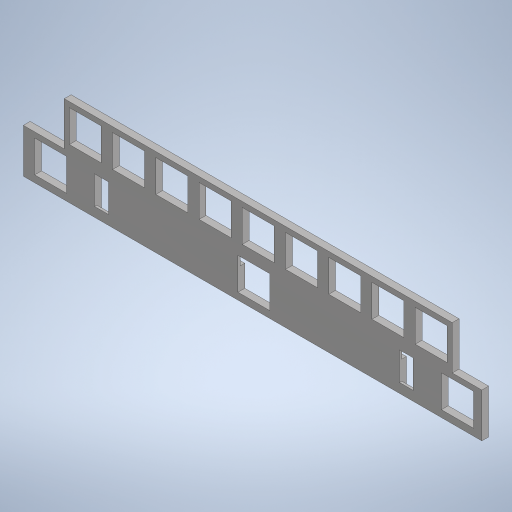
# Autodesk Inventor part: Lower Middle Plate
Saved by Autodesk Inventor 2024 (Build 280153000, 153)
## iProperties
Created: 2024-06-29
Part Number: Lower Middle Plate
Material: PET Plastic
Document SubType Name: Modeling
Designer: adam
Density: 1.541 g/cm^3
Appearance: Light Gray
Author: adam
Autodesk Inventor part; units mm, degrees
ref_plane "YZ Plane" through (0, 0, 0) normal (1, 0, 0) x (0, 1, 0)
ref_plane "XZ Plane" through (0, 0, 0) normal (0, 1, 0) x (-1, 0, 0)
ref_plane "XY Plane" through (0, 0, 0) normal (0, 0, 1) x (1, 0, 0)
sketch "Sketch1" plane through (0, 0, 0) normal (0, 0, 1) x (1, 0, 0)
  line L0 (31.275, 11.925) -> (31.275, -2.125) construction
  line L1 (31.275, -2.125) -> (17.225, -2.125) construction
  line L2 (17.225, -2.125) -> (17.225, 11.925) construction
  line L3 (17.225, 11.925) -> (31.275, 11.925) construction
  line L4 (-101.725, 11.925) -> (-101.725, -2.125) construction
  line L5 (-101.725, -2.125) -> (-115.775, -2.125) construction
  line L6 (-115.775, -2.125) -> (-115.775, 11.925) construction
  line L7 (-115.775, 11.925) -> (-101.725, 11.925) construction
  line L8 (43.325, -43.95) -> (49.375, -43.95) construction
  line L9 (49.375, -43.95) -> (49.375, -61) construction
  line L10 (49.375, -61) -> (43.325, -61) construction
  line L11 (43.325, -61) -> (43.325, -43.95) construction
  line L12 (117.95, -19.8) -> (117.95, -13.75) construction
  line L13 (117.95, -13.75) -> (135, -13.75) construction
  line L14 (135, -13.75) -> (135, -19.8) construction
  line L15 (135, -19.8) -> (117.95, -19.8) construction
  line L16 (26.325, -43.95) -> (32.375, -43.95) construction
  line L17 (32.375, -43.95) -> (32.375, -61) construction
  line L18 (32.375, -61) -> (26.325, -61) construction
  line L19 (26.325, -61) -> (26.325, -43.95) construction
  line L20 (-152.525, 13.425) -> (-146.475, 13.425) construction
  line L21 (-146.475, 13.425) -> (-146.475, -3.625) construction
  line L22 (-146.475, -3.625) -> (-152.525, -3.625) construction
  line L23 (-152.525, -3.625) -> (-152.525, 13.425) construction
  line L24 (-90.675, -43.95) -> (-84.625, -43.95) construction
  line L25 (-84.625, -43.95) -> (-84.625, -61) construction
  line L26 (-84.625, -61) -> (-90.675, -61) construction
  line L27 (-90.675, -61) -> (-90.675, -43.95) construction
  line L28 (39.375, -43.95) -> (39.375, -61) construction
  line L29 (39.375, -61) -> (33.325, -61) construction
  line L30 (33.325, -61) -> (33.325, -43.95) construction
  line L31 (33.325, -43.95) -> (39.375, -43.95) construction
  line L32 (117.95, 4.2) -> (117.95, 10.25) construction
  line L33 (117.95, 10.25) -> (135, 10.25) construction
  line L34 (135, 10.25) -> (135, 4.2) construction
  line L35 (135, 4.2) -> (117.95, 4.2) construction
  line L36 (-67.625, -43.95) -> (-67.625, -61) construction
  line L37 (-67.625, -61) -> (-73.675, -61) construction
  line L38 (-73.675, -61) -> (-73.675, -43.95) construction
  line L39 (-73.675, -43.95) -> (-67.625, -43.95) construction
  line L40 (-128.525, 13.425) -> (-122.475, 13.425) construction
  line L41 (-122.475, 13.425) -> (-122.475, -3.625) construction
  line L42 (-122.475, -3.625) -> (-128.525, -3.625) construction
  line L43 (-128.525, -3.625) -> (-128.525, 13.425) construction
  line L44 (-74.625, -43.95) -> (-74.625, -61) construction
  line L45 (-74.625, -61) -> (-80.675, -61) construction
  line L46 (-80.675, -61) -> (-80.675, -43.95) construction
  line L47 (-80.675, -43.95) -> (-74.625, -43.95) construction
  line L48 (-157.5, -62.5) -> (157.5, -62.5) construction
  line L49 (157.5, -62.5) -> (157.5, -41.5) construction
  line L50 (157.5, -41.5) -> (139.5, -41.5) construction
  line L51 (139.5, -41.5) -> (139.5, 12.5) construction
  line L52 (139.5, 12.5) -> (157.5, 12.5) construction
  line L53 (157.5, 12.5) -> (157.5, 62.5) construction
  line L54 (157.5, 62.5) -> (-157.5, 62.5) construction
  line L55 (-157.5, 62.5) -> (-157.5, -62.5) construction
  line L56 (-38.5, 42.5) -> (6.5, 42.5) construction
  line L57 (6.5, 42.5) -> (6.5, 33.5) construction
  line L58 (6.5, 33.5) -> (-38.5, 33.5) construction
  line L59 (-38.5, 33.5) -> (-38.5, 42.5) construction
  line L60 (154.775, -45.45) -> (154.775, -59.5) construction
  line L61 (154.775, -59.5) -> (140.725, -59.5) construction
  line L62 (140.725, -59.5) -> (140.725, -45.45) construction
  line L63 (140.725, -45.45) -> (154.775, -45.45) construction
  line L64 (135.775, -45.45) -> (135.775, -59.5) construction
  line L65 (135.775, -59.5) -> (121.725, -59.5) construction
  line L66 (121.725, -59.5) -> (121.725, -45.45) construction
  line L67 (121.725, -45.45) -> (135.775, -45.45) construction
  line L68 (116.775, -45.45) -> (116.775, -59.5) construction
  line L69 (116.775, -59.5) -> (102.725, -59.5) construction
  line L70 (102.725, -59.5) -> (102.725, -45.45) construction
  line L71 (102.725, -45.45) -> (116.775, -45.45) construction
  line L72 (97.775, -45.45) -> (97.775, -59.5) construction
  line L73 (97.775, -59.5) -> (83.725, -59.5) construction
  line L74 (83.725, -59.5) -> (83.725, -45.45) construction
  line L75 (83.725, -45.45) -> (97.775, -45.45) construction
  line L76 (75.775, -45.45) -> (75.775, -59.5) construction
  line L77 (75.775, -59.5) -> (61.725, -59.5) construction
  line L78 (61.725, -59.5) -> (61.725, -45.45) construction
  line L79 (61.725, -45.45) -> (75.775, -45.45) construction
  line L80 (-13.625, -45.45) -> (-13.625, -59.5) construction
  line L81 (-13.625, -59.5) -> (-27.675, -59.5) construction
  line L82 (-27.675, -59.5) -> (-27.675, -45.45) construction
  line L83 (-27.675, -45.45) -> (-13.625, -45.45) construction
  line L84 (-102.975, -45.45) -> (-102.975, -59.5) construction
  line L85 (-102.975, -59.5) -> (-117.025, -59.5) construction
  line L86 (-117.025, -59.5) -> (-117.025, -45.45) construction
  line L87 (-117.025, -45.45) -> (-102.975, -45.45) construction
  line L88 (-141.525, -45.45) -> (-127.475, -45.45) construction
  line L89 (-127.475, -45.45) -> (-127.475, -59.5) construction
  line L90 (-127.475, -59.5) -> (-141.525, -59.5) construction
  line L91 (-141.525, -59.5) -> (-141.525, -45.45) construction
  line L92 (121.725, -26.275) -> (135.775, -26.275) construction
  line L93 (135.775, -26.275) -> (135.775, -40.325) construction
  line L94 (135.775, -40.325) -> (121.725, -40.325) construction
  line L95 (121.725, -40.325) -> (121.725, -26.275) construction
  line L96 (95.475, -26.275) -> (109.525, -26.275) construction
  line L97 (109.525, -26.275) -> (109.525, -40.325) construction
  line L98 (109.525, -40.325) -> (95.475, -40.325) construction
  line L99 (95.475, -40.325) -> (95.475, -26.275) construction
  line L100 (69.225, -26.275) -> (83.275, -26.275) construction
  line L101 (83.275, -26.275) -> (83.275, -40.325) construction
  line L102 (83.275, -40.325) -> (69.225, -40.325) construction
  line L103 (69.225, -40.325) -> (69.225, -26.275) construction
  line L104 (50.225, -26.275) -> (64.275, -26.275) construction
  line L105 (64.275, -26.275) -> (64.275, -40.325) construction
  line L106 (64.275, -40.325) -> (50.225, -40.325) construction
  line L107 (50.225, -40.325) -> (50.225, -26.275) construction
  line L108 (31.225, -26.275) -> (45.275, -26.275) construction
  line L109 (45.275, -26.275) -> (45.275, -40.325) construction
  line L110 (45.275, -40.325) -> (31.225, -40.325) construction
  line L111 (31.225, -40.325) -> (31.225, -26.275) construction
  line L112 (12.225, -26.275) -> (26.275, -26.275) construction
  line L113 (26.275, -26.275) -> (26.275, -40.325) construction
  line L114 (26.275, -40.325) -> (12.225, -40.325) construction
  line L115 (12.225, -40.325) -> (12.225, -26.275) construction
  line L116 (-6.775, -26.275) -> (7.275, -26.275) construction
  line L117 (7.275, -26.275) -> (7.275, -40.325) construction
  line L118 (7.275, -40.325) -> (-6.775, -40.325) construction
  line L119 (-6.775, -40.325) -> (-6.775, -26.275) construction
  line L120 (-25.775, -26.275) -> (-11.725, -26.275) construction
  line L121 (-11.725, -26.275) -> (-11.725, -40.325) construction
  line L122 (-11.725, -40.325) -> (-25.775, -40.325) construction
  line L123 (-25.775, -40.325) -> (-25.775, -26.275) construction
  line L124 (-44.775, -26.275) -> (-30.725, -26.275) construction
  line L125 (-30.725, -26.275) -> (-30.725, -40.325) construction
  line L126 (-30.725, -40.325) -> (-44.775, -40.325) construction
  line L127 (-44.775, -40.325) -> (-44.775, -26.275) construction
  line L128 (-63.775, -26.275) -> (-49.725, -26.275) construction
  line L129 (-49.725, -26.275) -> (-49.725, -40.325) construction
  line L130 (-49.725, -40.325) -> (-63.775, -40.325) construction
  line L131 (-63.775, -40.325) -> (-63.775, -26.275) construction
  line L132 (-82.775, -26.275) -> (-68.725, -26.275) construction
  line L133 (-68.725, -26.275) -> (-68.725, -40.325) construction
  line L134 (-68.725, -40.325) -> (-82.775, -40.325) construction
  line L135 (-82.775, -40.325) -> (-82.775, -26.275) construction
  line L136 (-101.775, -26.275) -> (-87.725, -26.275) construction
  line L137 (-87.725, -26.275) -> (-87.725, -40.325) construction
  line L138 (-87.725, -40.325) -> (-101.775, -40.325) construction
  line L139 (-101.775, -40.325) -> (-101.775, -26.275) construction
  line L140 (-120.775, -26.275) -> (-106.725, -26.275) construction
  line L141 (-106.725, -26.275) -> (-106.725, -40.325) construction
  line L142 (-106.725, -40.325) -> (-120.775, -40.325) construction
  line L143 (-120.775, -40.325) -> (-120.775, -26.275) construction
  line L144 (-146.775, -26.275) -> (-132.725, -26.275) construction
  line L145 (-132.725, -26.275) -> (-132.725, -40.325) construction
  line L146 (-132.725, -40.325) -> (-146.775, -40.325) construction
  line L147 (-146.775, -40.325) -> (-146.775, -26.275) construction
  line L148 (97.975, -7.175) -> (112.025, -7.175) construction
  line L149 (112.025, -7.175) -> (112.025, -21.225) construction
  line L150 (112.025, -21.225) -> (97.975, -21.225) construction
  line L151 (97.975, -21.225) -> (97.975, -7.175) construction
  line L152 (78.975, -7.175) -> (93.025, -7.175) construction
  line L153 (93.025, -7.175) -> (93.025, -21.225) construction
  line L154 (93.025, -21.225) -> (78.975, -21.225) construction
  line L155 (78.975, -21.225) -> (78.975, -7.175) construction
  line L156 (59.975, -7.175) -> (74.025, -7.175) construction
  line L157 (74.025, -7.175) -> (74.025, -21.225) construction
  line L158 (74.025, -21.225) -> (59.975, -21.225) construction
  line L159 (59.975, -21.225) -> (59.975, -7.175) construction
  line L160 (40.975, -7.175) -> (55.025, -7.175) construction
  line L161 (55.025, -7.175) -> (55.025, -21.225) construction
  line L162 (55.025, -21.225) -> (40.975, -21.225) construction
  line L163 (40.975, -21.225) -> (40.975, -7.175) construction
  line L164 (21.975, -7.175) -> (36.025, -7.175) construction
  line L165 (36.025, -7.175) -> (36.025, -21.225) construction
  line L166 (36.025, -21.225) -> (21.975, -21.225) construction
  line L167 (21.975, -21.225) -> (21.975, -7.175) construction
  line L168 (2.975, -7.175) -> (17.025, -7.175) construction
  line L169 (17.025, -7.175) -> (17.025, -21.225) construction
  line L170 (17.025, -21.225) -> (2.975, -21.225) construction
  line L171 (2.975, -21.225) -> (2.975, -7.175) construction
  line L172 (-16.025, -7.175) -> (-1.975, -7.175) construction
  line L173 (-1.975, -7.175) -> (-1.975, -21.225) construction
  line L174 (-1.975, -21.225) -> (-16.025, -21.225) construction
  line L175 (-16.025, -21.225) -> (-16.025, -7.175) construction
  line L176 (-35.025, -7.175) -> (-20.975, -7.175) construction
  line L177 (-20.975, -7.175) -> (-20.975, -21.225) construction
  line L178 (-20.975, -21.225) -> (-35.025, -21.225) construction
  line L179 (-35.025, -21.225) -> (-35.025, -7.175) construction
  line L180 (-54.025, -7.175) -> (-39.975, -7.175) construction
  line L181 (-39.975, -7.175) -> (-39.975, -21.225) construction
  line L182 (-39.975, -21.225) -> (-54.025, -21.225) construction
  line L183 (-54.025, -21.225) -> (-54.025, -7.175) construction
  line L184 (-73.025, -7.175) -> (-58.975, -7.175) construction
  line L185 (-58.975, -7.175) -> (-58.975, -21.225) construction
  line L186 (-58.975, -21.225) -> (-73.025, -21.225) construction
  line L187 (-73.025, -21.225) -> (-73.025, -7.175) construction
  line L188 (-92.025, -7.175) -> (-77.975, -7.175) construction
  line L189 (-77.975, -7.175) -> (-77.975, -21.225) construction
  line L190 (-77.975, -21.225) -> (-92.025, -21.225) construction
  line L191 (-92.025, -21.225) -> (-92.025, -7.175) construction
  line L192 (-111.025, -7.175) -> (-96.975, -7.175) construction
  line L193 (-96.975, -7.175) -> (-96.975, -21.225) construction
  line L194 (-96.975, -21.225) -> (-111.025, -21.225) construction
  line L195 (-111.025, -21.225) -> (-111.025, -7.175) construction
  line L196 (-130.025, -7.175) -> (-115.975, -7.175) construction
  line L197 (-115.975, -7.175) -> (-115.975, -21.225) construction
  line L198 (-115.975, -21.225) -> (-130.025, -21.225) construction
  line L199 (-130.025, -21.225) -> (-130.025, -7.175) construction
  line L200 (-151.525, -7.175) -> (-137.475, -7.175) construction
  line L201 (-137.475, -7.175) -> (-137.475, -21.225) construction
  line L202 (-137.475, -21.225) -> (-151.525, -21.225) construction
  line L203 (-151.525, -21.225) -> (-151.525, -7.175) construction
  line L204 (119.45, 2.25) -> (133.5, 2.25) construction
  line L205 (133.5, 2.25) -> (133.5, -11.8) construction
  line L206 (133.5, -11.8) -> (119.45, -11.8) construction
  line L207 (119.45, -11.8) -> (119.45, 2.25) construction
  line L208 (107.275, 11.925) -> (107.275, -2.125) construction
  line L209 (107.275, -2.125) -> (93.225, -2.125) construction
  line L210 (93.225, -2.125) -> (93.225, 11.925) construction
  line L211 (93.225, 11.925) -> (107.275, 11.925) construction
  line L212 (88.275, 11.925) -> (88.275, -2.125) construction
  line L213 (88.275, -2.125) -> (74.225, -2.125) construction
  line L214 (74.225, -2.125) -> (74.225, 11.925) construction
  line L215 (74.225, 11.925) -> (88.275, 11.925) construction
  line L216 (69.275, 11.925) -> (69.275, -2.125) construction
  line L217 (69.275, -2.125) -> (55.225, -2.125) construction
  line L218 (55.225, -2.125) -> (55.225, 11.925) construction
  line L219 (55.225, 11.925) -> (69.275, 11.925) construction
  line L220 (50.275, 11.925) -> (50.275, -2.125) construction
  line L221 (50.275, -2.125) -> (36.225, -2.125) construction
  line L222 (36.225, -2.125) -> (36.225, 11.925) construction
  line L223 (36.225, 11.925) -> (50.275, 11.925) construction
  line L224 (12.275, 11.925) -> (12.275, -2.125) construction
  line L225 (12.275, -2.125) -> (-1.775, -2.125) construction
  line L226 (-1.775, -2.125) -> (-1.775, 11.925) construction
  line L227 (-1.775, 11.925) -> (12.275, 11.925) construction
  line L228 (-6.725, 11.925) -> (-6.725, -2.125) construction
  line L229 (-6.725, -2.125) -> (-20.775, -2.125) construction
  line L230 (-20.775, -2.125) -> (-20.775, 11.925) construction
  line L231 (-20.775, 11.925) -> (-6.725, 11.925) construction
  line L232 (-25.725, 11.925) -> (-25.725, -2.125) construction
  line L233 (-25.725, -2.125) -> (-39.775, -2.125) construction
  line L234 (-39.775, -2.125) -> (-39.775, 11.925) construction
  line L235 (-39.775, 11.925) -> (-25.725, 11.925) construction
  line L236 (-44.725, 11.925) -> (-44.725, -2.125) construction
  line L237 (-44.725, -2.125) -> (-58.775, -2.125) construction
  line L238 (-58.775, -2.125) -> (-58.775, 11.925) construction
  line L239 (-58.775, 11.925) -> (-44.725, 11.925) construction
  line L240 (-63.725, 11.925) -> (-63.725, -2.125) construction
  line L241 (-63.725, -2.125) -> (-77.775, -2.125) construction
  line L242 (-77.775, -2.125) -> (-77.775, 11.925) construction
  line L243 (-77.775, 11.925) -> (-63.725, 11.925) construction
  line L244 (-82.725, 11.925) -> (-82.725, -2.125) construction
  line L245 (-82.725, -2.125) -> (-96.775, -2.125) construction
  line L246 (-96.775, -2.125) -> (-96.775, 11.925) construction
  line L247 (-96.775, 11.925) -> (-82.725, 11.925) construction
  line L248 (-144.525, 11.925) -> (-130.475, 11.925) construction
  line L249 (-130.475, 11.925) -> (-130.475, -2.125) construction
  line L250 (-130.475, -2.125) -> (-144.525, -2.125) construction
  line L251 (-144.525, -2.125) -> (-144.525, 11.925) construction
  line L252 (154.525, 16.975) -> (140.475, 16.975) construction
  line L253 (140.475, 16.975) -> (140.475, 31.025) construction
  line L254 (140.475, 31.025) -> (154.525, 31.025) construction
  line L255 (154.525, 31.025) -> (154.525, 16.975) construction
  line L256 (135.525, 16.975) -> (121.475, 16.975) construction
  line L257 (121.475, 16.975) -> (121.475, 31.025) construction
  line L258 (121.475, 31.025) -> (135.525, 31.025) construction
  line L259 (135.525, 31.025) -> (135.525, 16.975) construction
  line L260 (116.525, 16.975) -> (102.475, 16.975) construction
  line L261 (102.475, 16.975) -> (102.475, 31.025) construction
  line L262 (102.475, 31.025) -> (116.525, 31.025) construction
  line L263 (116.525, 31.025) -> (116.525, 16.975) construction
  line L264 (97.525, 16.975) -> (83.475, 16.975) construction
  line L265 (83.475, 16.975) -> (83.475, 31.025) construction
  line L266 (83.475, 31.025) -> (97.525, 31.025) construction
  line L267 (97.525, 31.025) -> (97.525, 16.975) construction
  line L268 (78.525, 16.975) -> (64.475, 16.975) construction
  line L269 (64.475, 16.975) -> (64.475, 31.025) construction
  line L270 (64.475, 31.025) -> (78.525, 31.025) construction
  line L271 (78.525, 31.025) -> (78.525, 16.975) construction
  line L272 (59.525, 16.975) -> (45.475, 16.975) construction
  line L273 (45.475, 16.975) -> (45.475, 31.025) construction
  line L274 (45.475, 31.025) -> (59.525, 31.025) construction
  line L275 (59.525, 31.025) -> (59.525, 16.975) construction
  line L276 (40.525, 16.975) -> (26.475, 16.975) construction
  line L277 (26.475, 16.975) -> (26.475, 31.025) construction
  line L278 (26.475, 31.025) -> (40.525, 31.025) construction
  line L279 (40.525, 31.025) -> (40.525, 16.975) construction
  line L280 (21.525, 16.975) -> (7.475, 16.975) construction
  line L281 (7.475, 16.975) -> (7.475, 31.025) construction
  line L282 (7.475, 31.025) -> (21.525, 31.025) construction
  line L283 (21.525, 31.025) -> (21.525, 16.975) construction
  line L284 (2.525, 16.975) -> (-11.525, 16.975) construction
  line L285 (-11.525, 16.975) -> (-11.525, 31.025) construction
  line L286 (-11.525, 31.025) -> (2.525, 31.025) construction
  line L287 (2.525, 31.025) -> (2.525, 16.975) construction
  line L288 (-16.475, 16.975) -> (-30.525, 16.975) construction
  line L289 (-30.525, 16.975) -> (-30.525, 31.025) construction
  line L290 (-30.525, 31.025) -> (-16.475, 31.025) construction
  line L291 (-16.475, 31.025) -> (-16.475, 16.975) construction
  line L292 (-35.475, 16.975) -> (-49.525, 16.975) construction
  line L293 (-49.525, 16.975) -> (-49.525, 31.025) construction
  line L294 (-49.525, 31.025) -> (-35.475, 31.025) construction
  line L295 (-35.475, 31.025) -> (-35.475, 16.975) construction
  line L296 (-54.475, 16.975) -> (-68.525, 16.975) construction
  line L297 (-68.525, 16.975) -> (-68.525, 31.025) construction
  line L298 (-68.525, 31.025) -> (-54.475, 31.025) construction
  line L299 (-54.475, 31.025) -> (-54.475, 16.975) construction
  line L300 (-73.475, 16.975) -> (-87.525, 16.975) construction
  line L301 (-87.525, 16.975) -> (-87.525, 31.025) construction
  line L302 (-87.525, 31.025) -> (-73.475, 31.025) construction
  line L303 (-73.475, 31.025) -> (-73.475, 16.975) construction
  line L304 (-92.475, 16.975) -> (-106.525, 16.975) construction
  line L305 (-106.525, 16.975) -> (-106.525, 31.025) construction
  line L306 (-106.525, 31.025) -> (-92.475, 31.025) construction
  line L307 (-92.475, 31.025) -> (-92.475, 16.975) construction
  line L308 (-111.475, 16.975) -> (-125.525, 16.975) construction
  line L309 (-125.525, 16.975) -> (-125.525, 31.025) construction
  line L310 (-125.525, 31.025) -> (-111.475, 31.025) construction
  line L311 (-111.475, 31.025) -> (-111.475, 16.975) construction
  line L312 (-149.525, 31.025) -> (-135.475, 31.025) construction
  line L313 (-135.475, 31.025) -> (-135.475, 16.975) construction
  line L314 (-135.475, 16.975) -> (-149.525, 16.975) construction
  line L315 (-149.525, 16.975) -> (-149.525, 31.025) construction
  line L316 (138.975, 59.525) -> (153.025, 59.525) construction
  line L317 (153.025, 59.525) -> (153.025, 45.475) construction
  line L318 (153.025, 45.475) -> (138.975, 45.475) construction
  line L319 (138.975, 45.475) -> (138.975, 59.525) construction
  line L320 (105.475, 59.525) -> (119.525, 59.525) construction
  line L321 (119.525, 59.525) -> (119.525, 45.475) construction
  line L322 (119.525, 45.475) -> (105.475, 45.475) construction
  line L323 (105.475, 45.475) -> (105.475, 59.525) construction
  line L324 (81.475, 59.525) -> (95.525, 59.525) construction
  line L325 (95.525, 59.525) -> (95.525, 45.475) construction
  line L326 (95.525, 45.475) -> (81.475, 45.475) construction
  line L327 (81.475, 45.475) -> (81.475, 59.525) construction
  line L328 (57.475, 59.525) -> (71.525, 59.525) construction
  line L329 (71.525, 59.525) -> (71.525, 45.475) construction
  line L330 (71.525, 45.475) -> (57.475, 45.475) construction
  line L331 (57.475, 45.475) -> (57.475, 59.525) construction
  line L332 (33.475, 59.525) -> (47.525, 59.525) construction
  line L333 (47.525, 59.525) -> (47.525, 45.475) construction
  line L334 (47.525, 45.475) -> (33.475, 45.475) construction
  line L335 (33.475, 45.475) -> (33.475, 59.525) construction
  line L336 (9.475, 59.525) -> (23.525, 59.525) construction
  line L337 (23.525, 59.525) -> (23.525, 45.475) construction
  line L338 (23.525, 45.475) -> (9.475, 45.475) construction
  line L339 (9.475, 45.475) -> (9.475, 59.525) construction
  line L340 (-23.025, 59.525) -> (-8.975, 59.525) construction
  line L341 (-8.975, 59.525) -> (-8.975, 45.475) construction
  line L342 (-8.975, 45.475) -> (-23.025, 45.475) construction
  line L343 (-23.025, 45.475) -> (-23.025, 59.525) construction
  line L344 (-47.025, 59.525) -> (-32.975, 59.525) construction
  line L345 (-32.975, 59.525) -> (-32.975, 45.475) construction
  line L346 (-32.975, 45.475) -> (-47.025, 45.475) construction
  line L347 (-47.025, 45.475) -> (-47.025, 59.525) construction
  line L348 (-71.025, 59.525) -> (-56.975, 59.525) construction
  line L349 (-56.975, 59.525) -> (-56.975, 45.475) construction
  line L350 (-56.975, 45.475) -> (-71.025, 45.475) construction
  line L351 (-71.025, 45.475) -> (-71.025, 59.525) construction
  line L352 (-95.025, 59.525) -> (-80.975, 59.525) construction
  line L353 (-80.975, 59.525) -> (-80.975, 45.475) construction
  line L354 (-80.975, 45.475) -> (-95.025, 45.475) construction
  line L355 (-95.025, 45.475) -> (-95.025, 59.525) construction
  line L356 (-119.025, 59.525) -> (-104.975, 59.525) construction
  line L357 (-104.975, 59.525) -> (-104.975, 45.475) construction
  line L358 (-104.975, 45.475) -> (-119.025, 45.475) construction
  line L359 (-119.025, 45.475) -> (-119.025, 59.525) construction
  line L360 (-152.025, 59.525) -> (-137.975, 59.525) construction
  line L361 (-137.975, 59.525) -> (-137.975, 45.475) construction
  line L362 (-137.975, 45.475) -> (-152.025, 45.475) construction
  line L363 (-152.025, 45.475) -> (-152.025, 59.525) construction
  line L364 (-122.25, -62.5) -> (-122.25, -42.8875) construction
  line L365 (-122.25, -42.8875) -> (-104.25, -42.8875) construction
  line L366 (-104.25, -42.8875) -> (-104.25, -23.75) construction
  line L367 (-104.25, -23.75) -> (66.75, -23.75) construction
  line L368 (66.75, -23.75) -> (66.75, -42.8875) construction
  line L369 (66.75, -42.8875) -> (79.75, -42.8875) construction
  line L370 (79.75, -42.8875) -> (79.75, -62.5) construction
  line L371 (75.775, -45.45) -> (79.75, -45.45) construction
  line L372 (79.75, -45.45) -> (83.725, -45.45) construction
  line L373 (75.775, -45.45) -> (75.775, -42.8875) construction
  line L374 (75.775, -42.8875) -> (75.775, -40.325) construction
  line L375 (69.225, -40.325) -> (66.75, -40.325) construction
  line L376 (66.75, -40.325) -> (64.275, -40.325) construction
  line L377 (64.275, -26.275) -> (64.275, -23.75) construction
  line L378 (64.275, -23.75) -> (64.275, -21.225) construction
  line L379 (-106.725, -26.275) -> (-104.25, -26.275) construction
  line L380 (-104.25, -26.275) -> (-101.775, -26.275) construction
  line L381 (-106.725, -40.325) -> (-106.725, -42.8875) construction
  line L382 (-106.725, -42.8875) -> (-106.725, -45.45) construction
  line L383 (-127.475, -45.45) -> (-122.25, -45.45) construction
  line L384 (-122.25, -45.45) -> (-117.025, -45.45) construction
  line L385 (-122, -62.5) -> (-122, -43.1375)
  line L386 (-122, -43.1375) -> (-104, -43.1375)
  line L387 (-104, -43.1375) -> (-104, -24)
  line L388 (-104, -24) -> (66.5, -24)
  line L389 (66.5, -24) -> (66.5, -43.1375)
  line L390 (66.5, -43.1375) -> (79.5, -43.1375)
  line L391 (79.5, -43.1375) -> (79.5, -62.5)
  line L392 (79.5, -62.5) -> (-122, -62.5)
  line L393 (-102.975, -45.45) -> (-102.975, -59.5) projected
  line L394 (-117.025, -45.45) -> (-102.975, -45.45) projected
  line L395 (-117.025, -59.5) -> (-117.025, -45.45) projected
  line L396 (-102.975, -59.5) -> (-117.025, -59.5) projected
  line L397 (-87.725, -40.325) -> (-101.775, -40.325) projected
  line L398 (-101.775, -40.325) -> (-101.775, -26.275) projected
  line L399 (-101.775, -26.275) -> (-87.725, -26.275) projected
  line L400 (-87.725, -26.275) -> (-87.725, -40.325) projected
  line L401 (-82.775, -40.325) -> (-82.775, -26.275) projected
  line L402 (-82.775, -26.275) -> (-68.725, -26.275) projected
  line L403 (-68.725, -26.275) -> (-68.725, -40.325) projected
  line L404 (-68.725, -40.325) -> (-82.775, -40.325) projected
  line L405 (-49.725, -40.325) -> (-63.775, -40.325) projected
  line L406 (-63.775, -40.325) -> (-63.775, -26.275) projected
  line L407 (-49.725, -26.275) -> (-49.725, -40.325) projected
  line L408 (-63.775, -26.275) -> (-49.725, -26.275) projected
  line L409 (-44.775, -40.325) -> (-44.775, -26.275) projected
  line L410 (-44.775, -26.275) -> (-30.725, -26.275) projected
  line L411 (-30.725, -40.325) -> (-44.775, -40.325) projected
  line L412 (-30.725, -26.275) -> (-30.725, -40.325) projected
  line L413 (-25.775, -26.275) -> (-11.725, -26.275) projected
  line L414 (-25.775, -40.325) -> (-25.775, -26.275) projected
  line L415 (-11.725, -26.275) -> (-11.725, -40.325) projected
  line L416 (-11.725, -40.325) -> (-25.775, -40.325) projected
  line L417 (-27.675, -45.45) -> (-13.625, -45.45) projected
  line L418 (-13.625, -45.45) -> (-13.625, -59.5) projected
  line L419 (-27.675, -59.5) -> (-27.675, -45.45) projected
  line L420 (-13.625, -59.5) -> (-27.675, -59.5) projected
  line L421 (-6.775, -40.325) -> (-6.775, -26.275) projected
  line L422 (7.275, -40.325) -> (-6.775, -40.325) projected
  line L423 (7.275, -26.275) -> (7.275, -40.325) projected
  line L424 (-6.775, -26.275) -> (7.275, -26.275) projected
  line L425 (12.225, -40.325) -> (12.225, -26.275) projected
  line L426 (12.225, -26.275) -> (26.275, -26.275) projected
  line L427 (26.275, -26.275) -> (26.275, -40.325) projected
  line L428 (26.275, -40.325) -> (12.225, -40.325) projected
  line L429 (31.225, -26.275) -> (45.275, -26.275) projected
  line L430 (45.275, -26.275) -> (45.275, -40.325) projected
  line L431 (31.225, -40.325) -> (31.225, -26.275) projected
  line L432 (45.275, -40.325) -> (31.225, -40.325) projected
  line L433 (50.225, -26.275) -> (64.275, -26.275) projected
  line L434 (50.225, -40.325) -> (50.225, -26.275) projected
  line L435 (64.275, -40.325) -> (50.225, -40.325) projected
  line L436 (64.275, -26.275) -> (64.275, -40.325) projected
  line L437 (61.725, -45.45) -> (75.775, -45.45) projected
  line L438 (75.775, -45.45) -> (75.775, -59.5) projected
  line L439 (61.725, -59.5) -> (61.725, -45.45) projected
  line L440 (75.775, -59.5) -> (61.725, -59.5) projected
  line L441 (-90.675, -45.95) -> (-84.625, -45.95)
  line L442 (-90.675, -58.35) -> (-84.625, -58.35)
  line L443 (-90.675, -45.95) -> (-90.675, -58.35)
  line L444 (-84.625, -45.95) -> (-84.625, -58.35)
  line L445 (43.325, -45.95) -> (49.375, -45.95)
  line L446 (43.325, -58.35) -> (49.375, -58.35)
  line L447 (43.325, -45.95) -> (43.325, -58.35)
  line L448 (49.375, -45.95) -> (49.375, -58.35)
  point P0 (0, 0)
  dimension "d0" = 0.25
  dimension "d1" = 0.25
  dimension "d2" = 0.25
  dimension "d3" = 0.25
  dimension "d4" = 0.25
  dimension "d5" = 0.25
  dimension "d6" = 0.25
  dimension "d7" = 2
  dimension "d8" = 12.4
  constraints: 74 end point, 26 point on line, 21 perpendicular, 17 collinear, 2 parallel, 2 vertical
  measures "d0" distance between parallel lines of L385 L364
  measures "d1" distance between parallel lines of L386 L365
  measures "d2" distance between parallel lines of L387 L366
  measures "d3" distance between parallel lines of L388 L367
  measures "d4" distance between parallel lines of L368 L389
  measures "d5" distance between parallel lines of L390 L369
  measures "d6" distance between parallel lines of L370 L391
  measures "d7" distance between parallel lines of L24 L441
  measures "d8" distance between parallel lines of L442 L441
extrude "Extrusion1" add sketch "Sketch1" along normal blind 3
sketch "Sketch2" plane through (0, 0, 0) normal (0, 0, -1) x (-1, 0, 0)
  line L0 (-49.375, -60.35) -> (-43.325, -60.35)
  line L1 (-43.325, -60.35) -> (-43.325, -49.95)
  line L2 (-43.325, -42.95) -> (-49.375, -42.95)
  line L3 (-49.375, -42.95) -> (-49.375, -60.35)
  line L4 (-43.325, -45.95) -> (-49.375, -45.95) projected
  line L5 (-49.375, -61) -> (-49.375, -43.95) construction
  line L6 (-43.325, -43.95) -> (-43.325, -61) construction
  line L7 (84.625, -61) -> (84.625, -43.95) construction
  line L8 (90.675, -43.95) -> (90.675, -61) construction
  line L9 (84.625, -42.95) -> (90.675, -42.95)
  line L10 (90.675, -42.95) -> (90.675, -60.35)
  line L11 (90.675, -60.35) -> (84.625, -60.35)
  line L12 (84.625, -60.35) -> (84.625, -49.95)
  line L13 (-43.325, -42.95) -> (84.625, -42.95)
  line L14 (-43.325, -49.95) -> (84.625, -49.95)
  line L15 (84.625, -45.95) -> (84.625, -58.35) projected
  point P0 (0, 0)
  point P1 (-49.375, -58.35)
  point P2 (-43.325, -58.35)
  dimension "d12" = 3
  dimension "d13" = 4
  constraints: 20 end point, 6 collinear, 4 parallel, 3 perpendicular, 3 point on line, 2 horizontal
  measures "d12" distance between parallel lines of L2 L4
  measures "d13" distance between parallel lines of L14 L4
extrude "Extrusion2" cut sketch "Sketch2" against normal blind 2
equation "\"d0\" = ipg"
equation "\"d1\" = ipg"
equation "\"d2\" = ipg"
equation "\"d3\" = ipg"
equation "\"d4\" = ipg"
equation "\"d5\" = ipg"
equation "\"d6\" = ipg"
equation "\"ipg\" = 0.25"
body "Solid1"
